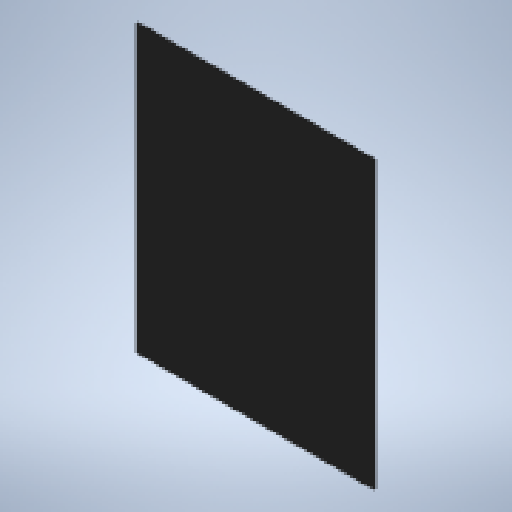
# Autodesk Inventor part: Bed Magnet
Saved by Autodesk Inventor 2024 (Build 280153000, 153)
## iProperties
Created: 2024-08-02
Part Number: Bed Magnet
Material: Acetal Resin, Black
Document SubType Name: Modeling
Designer: Ishaan
Density: 1.425 g/cm^3
Appearance: Smooth - Black
Author: Ishaan
Autodesk Inventor part; units mm, degrees
ref_plane "YZ Plane" through (0, 0, 0) normal (1, 0, 0) x (0, 1, 0)
ref_plane "XZ Plane" through (0, 0, 0) normal (0, 1, 0) x (-1, 0, 0)
ref_plane "XY Plane" through (0, 0, 0) normal (0, 0, 1) x (1, 0, 0)
sketch "Sketch1" plane through (0, 0, 0) normal (0, 0, 1) x (1, 0, 0)
  line L0 (125, -150) -> (-125, -150)
  line L1 (-125, -150) -> (-125, 150)
  line L2 (-125, 150) -> (125, 150)
  line L3 (125, 150) -> (125, -150)
  line L4 (125, -150) -> (-125, 150) construction
  line L5 (-125, -150) -> (125, 150) construction
  point P0 (0, 0)
  dimension "d0" = 250
  dimension "d1" = 300
  constraints: 12 end point, 2 midpoint, 2 parallel, 1 horizontal, 1 perpendicular
  measures "d0" distance of L1.end L2.end
  measures "d1" distance of L0.end L1.end
extrude "Extrusion1" add sketch "Sketch1" along normal blind 1.5
body "Solid1"
